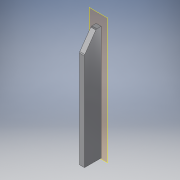
# Autodesk Inventor part: ZcolStiffer
Saved by Autodesk Inventor 2019 (Build 230136000, 136)
## iProperties
Created: 2018-10-03
Part Number: ZcolStiffer
Material: Aluminum 6061-AHC
Document SubType Name: Modeling
Designer: LillaHunden
Density: 2.7 g/cm^3
Appearance: Aluminum - Dark
Mass: 652.96 g
Surface Area: 435.759 cm^2
Volume: 241.837 cm^3
Author: LillaHunden
Autodesk Inventor part; units mm, degrees
ref_plane "YZ Plane" through (0, 0, 0) normal (1, 0, 0) x (0, 1, 0)
ref_plane "XZ Plane" through (0, 0, 0) normal (0, 1, 0) x (-1, 0, 0)
ref_plane "XY Plane" through (0, 0, 0) normal (0, 0, 1) x (1, 0, 0)
ref_plane "Work Plane1" through (0, 0, 0) normal (0, 0, 1) x (1, 0, 0)
sketch "Sketch1" plane through (0, 0, 0) normal (0, 0, 1) x (1, 0, 0)
  line L0 (1.0143, 326.2667) -> (51.0143, 326.2667) construction
  line L1 (0, -13.7333) -> (51.0143, -13.7333) construction
  line L2 (18.5143, 326.2667) -> (33.5143, 326.2667)
  line L3 (33.5143, 326.2667) -> (33.5143, -13.7333)
  line L4 (33.5143, -13.7333) -> (18.5143, -13.7333)
  line L5 (18.5143, -13.7333) -> (18.5143, 326.2667)
  point P0 (0, 0)
  point P1 (51.0143, -13.7333)
  point P2 (26.0143, 326.2667)
  point P3 (26.0143, 326.2667)
  dimension "d0" = 15
  constraints: 8 end point, 2 midpoint, 2 parallel, 1 coincident, 1 horizontal, 1 perpendicular, 1 point on line, 2 other
  measures "d0" distance of L3.end L4.end
extrude "Extrusion1" add sketch "Sketch1" along normal blind 50
sketch "Sketch2" plane through (33.5143, -13.7333, 0) normal (1, 0, 0) x (0, 0, -1)
  line L0 (0, 340) -> (-50, 340) projected
  line L1 (-15, 340) -> (-50, 290.0148)
  line L2 (-50, 0) -> (-50, 340) projected
  line L3 (0, 340) -> (0, 0) projected
  point P0 (0, 13.7333)
  dimension "d3" = 35
  dimension "d4" = 15
  constraints: 2 end point, 2 point on line
  measures "d3" angle of L2 L1
  measures "d4" distance from line of L1.start L3
extrude "Extrusion2" cut sketch "Sketch2" against normal through all
chamfer "Chamfer1" distance 2 angle 45 1 edges at (26.0143, 326.2667, 15)
chamfer "Chamfer2" distance 2 angle 45 1 edges at (26.0143, 276.2815, 50)
body "Solid1"
